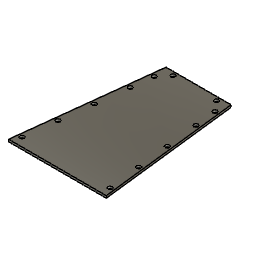
Basket Side v0 (1) (Autodesk Fusion 360 design; units mm, degrees)
Autodesk Fusion 360 part; units mm, degrees
sketch "Sketch1" plane through (0, 0, 0) normal (0, 0, 1) x (1, 0, 0)
  line L0 (0, 0) -> (60, 0)
  line L1 (30, 0) -> (30, -130)
  line L2 (30, -130) -> (75, -130)
  line L3 (30, -130) -> (-15, -130)
  line L4 (0, 0) -> (-15, -130)
  line L5 (60, 0) -> (75, -130)
  dimension "d1" = 60
  dimension "d2" = 130
  dimension "d3" = 45
  dimension "d4" = 45
  constraint coincident L0.start L4.start
  constraint horizontal L0
  constraint midpoint L0 L1.start
  constraint perpendicular L0 L1
  constraint perpendicular L1 L2
  constraint perpendicular L1 L3
  measures "d1" distance of L0.start L0.end
  measures "d2" distance of L1.start L1.end
  measures "d3" distance of L1.end L2.end
  measures "d4" distance of L1.end L3.end
extrude "Extrude1" add sketch "Sketch1" along normal blind 2
sketch "Sketch2" plane through (0, 0, 2) normal (0, 0, 1) x (-1, 0, 0)
  line L0 (0, 0) -> (15, 130)
  line L1 (15, 130) -> (-75, 130)
  line L2 (-75, 130) -> (-60, 0)
  line L3 (-60, 0) -> (0, 0)
  line L4 (-30, 0) -> (-30, 3.5)
  line L5 (-60, 0) -> (-50, 0)
  line L6 (-50, 0) -> (-50, 3.5)
  line L7 (-30, 0) -> (-30, 130)
  line L8 (-62.991, 25.9222) -> (-59.5141, 26.3233)
  line L9 (-64.2385, 36.7338) -> (-60.7616, 37.135)
  line L10 (-59.5141, 26.3233) -> (-71.4768, 130)
  line L11 (-60.7616, 37.135) -> (-56.4649, 0)
  line L12 (-60.7616, 37.135) -> (-23.3789, 37.135) construction
  line L13 (-71.4768, 130) -> (-70.5598, 122.0527)
  line L14 (-70.5598, 122.0527) -> (-67.1211, 92.2505)
  line L15 (-67.1211, 92.2505) -> (-63.6823, 62.4482)
  line L16 (-63.6823, 62.4482) -> (-60.2436, 32.6459)
  line L17 (-60.2436, 32.6459) -> (-57.9511, 12.7777)
  point P0 (11.4768, 130)
  point P1 (10.5598, 122.0527)
  point P2 (7.1211, 92.2505)
  point P3 (3.6823, 62.4482)
  point P4 (0.2436, 32.6459)
  point P5 (-2.0489, 12.7777)
  point P6 (-10, 3.5)
  dimension "d7" = 3.5
  dimension "d8" = 10
  dimension "d9" = 3.5
  dimension "d10" = 3.5
  dimension "d11" = 3.5
  dimension "d12" = 83.4
  dimension "d13" = 8
  dimension "d14" = 30
  dimension "d15" = 30
  dimension "d16" = 30
  dimension "d17" = 20
  constraint midpoint L3 L4.start
  constraint vertical L4
  constraint coincident L2.end L3.start
  constraint perpendicular L4 L5
  constraint perpendicular L5 L6
  constraint midpoint L1 L7.end
  constraint coincident L2 L8.start
  constraint perpendicular L2 L8
  constraint coincident L2 L9.start
  constraint perpendicular L2 L9
  constraint coincident L1 L10.end
  constraint perpendicular L9 L10
  constraint horizontal L12
  constraint coincident L3 L11.end
  constraint parallel L10 L13
  constraint coincident L10 L14.end
  constraint parallel L10 L15
  constraint perpendicular L9 L16
  constraint perpendicular L8 L17
  constraint symmetric L6.end L7 P6
  constraint symmetric L7 L10.end P0
  constraint symmetric L7 L13.end P1
  constraint symmetric L7 L14.end P2
  constraint symmetric L7 L15.end P3
  constraint symmetric L7 L16.end P4
  constraint symmetric L7 L17.end P5
  measures "d7" distance of L4.start L4.end
  measures "d8" distance of L2.end L5.end
  measures "d9" distance of L5.end L6.end
  measures "d10" distance of L8.start L8.end
  measures "d11" distance of L9.start L9.end
  measures "d12" angle of L11 L12
  measures "d13" distance of L10.end L13.end
  measures "d14" distance of L13.end L14.end
  measures "d15" distance of L14.end L15.end
  measures "d16" distance of L15.end L16.end
  measures "d17" distance of L16.end L17.end
hole "Hole1" at (10, -3.5, 2) at (2.0489, -12.7777, 2) at (-0.2436, -32.6459, 2) at (-3.6823, -62.4482, 2) at (-7.1211, -92.2505, 2) at (-10.5598, -122.0527, 2) at (50, -3.5, 2) at (57.9511, -12.7777, 2) at (63.6823, -62.4482, 2) at (67.1211, -92.2505, 2) at (70.5598, -122.0527, 2) at (60.2436, -32.6459, 2) direction (0, 0, -1) diameter 4 depth 50 tip angle 180
